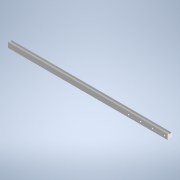
# Autodesk Inventor part: HSR35R128020 Rail
Saved by Autodesk Inventor 2022 (Build 260153000, 153)
## iProperties
Part Number: HSR35R128020 Rail
Material: Generic
Catalog Web Link: www.cadenas.de
Description: Compact Type - Heavy Load HSR-R Rail-Rail
Vendor: THK
Document SubType Name: Modeling
Designer: partserver
Manufacturer: THK
Mass: 224.938 g
Surface Area: 416.736 cm^2
Volume: 224.938 cm^3
Density: 1 g/cm^3
Appearance: PSOLRGB-192-192-192
Category: PARTsolutions
Company: THK
PSOL_IDENT_0: {$CADENAS_DATA\23d-libs\thk\linear_motion_systems\lm_guide\lm_guide\lm_guide_hsr\four_taped_hole_typ
PSOL_IDENT_1: e\hsr_r\hsr_r_rail.prj},219 {VTYP=3D},{NB=HSR35R128020 Rail},{LINA=HSR35R128020 Rail},{NN=Compact Ty
PSOL_IDENT_2: pe - Heavy Load HSR-R Rail},{DATE=21.06.2021 00:23:41},{GEOMDATE=24.12.2019 02:38:19},{VERSION=},{LI
PSOL_IDENT_3: NEID=70},{WBVAR=L,G,GX,TAPH},{WBNUMERIC=L,GX}  {NB=HSR35R128020 Rail},{LINA=HSR35R128020 Rail},{KT=D
PSOL_IDENT_4: UMMY},{MN=HSR35R},{NOB=1},{L=280.0},{G=},{GG='', 'Symmetrical (G1=G2)', 'A', 'Asymmetrical'},{GX=20}
PSOL_IDENT_5: ,{TAPH=},{GX1=20},{LMIN=109.4},{LEND=8640.00},{LMING=8.00},{LMAXG=32.00},{W1=34.00},{M1=29.00},{F=80
PSOL_IDENT_6: .00},{D1=9.00},{D2=14.00},{HM=12.00},{MAXL=3000.00},{GMIN=8},{GMX=20},{GMAX1=3.3},{G1=20},{G2=20},{N
PSOL_IDENT_7: X=1},{H3=7.50},{A=4},{LF=-20},{LM=320},{LL=620},{AA=3},{GMAX=32},{P=4},{PX=0},{VG=3},{VGG=20},{VG1=-
PSOL_IDENT_8: 1},{VG2=4},{ND=5.000},{LT=2880},{GA=20.000},{X=0.000},{S1=8.000},{L1=17.000},{NOTE=MIN}
NB: HSR35R128020 Rail
NN: Compact Type - Heavy Load HSR-R Rail
NT: Rail
NBSYN: $MN.$NOB.$L.$G.$GX.$TAPH. Rail
LINA: HSR35R128020 Rail
CATALOG: THK
MN: HSR35R
NOB: 1
L: 280
G: Symmetrical (G1=G2)
GX: 20
TAPH: Standard
LEND: 8640
LMING: 8
LMAXG: 32
W1: 34
M1: 29
F: 80
D1: 9
D2: 14
HM: 12
MAXL: 3000
H3: 7.5
ND: 5
GA: 20
X: 0
S1: 8
L1: 17
NOTE: 0
SUPPLIER: THK
ARTICLENO: HSR35R128020 Rail
BOMINFO: HSR35R128020 Rail
CREATOR: CADENAS GmbH
Title: HSR35R128020 Rail
Author: Cadenas PARTsolutions
Comments: Rail
Autodesk Inventor part; units mm, degrees
sketch "Sketch_18" plane through (-20, 0, 0) normal (1, 0, 0) x (0, 0, -1)
  line L0 (-17, 1.5) -> (-15.5, 0)
  line L1 (-15.5, 0) -> (-8.745, 0)
  line L2 (-8.745, 0) -> (-8.245, 0.5)
  line L3 (-8.245, 0.5) -> (-3.75, 0.5)
  line L4 (-3.75, 0.5) -> (-3.25, 0)
  line L5 (-3.25, 0) -> (3.25, 0)
  line L6 (3.25, 0) -> (3.75, 0.5)
  line L7 (3.75, 0.5) -> (8.245, 0.5)
  line L8 (8.245, 0.5) -> (8.745, 0)
  line L9 (8.745, 0) -> (15.5, 0)
  line L10 (15.5, 0) -> (17, 1.5)
  line L11 (17, 1.5) -> (17, 7.0002)
  line L12 (17, 7.0002) -> (11.8003, 12.1999)
  line L13 (11.8003, 12.1999) -> (11.8003, 17.6796)
  line L14 (11.8003, 17.6796) -> (13.6381, 19.5174)
  arc A0 (16.4816, 22.3609) -> (13.6381, 19.5174) centre (16.9102, 19.0889) ccw
  line L15 (16.4816, 22.3609) -> (17, 22.8793)
  line L16 (17, 22.8793) -> (17, 25.1102)
  line L17 (17, 25.1102) -> (16.4686, 25.6415)
  arc A1 (13.6398, 28.4703) -> (16.4686, 25.6415) centre (16.9102, 28.9119) ccw
  line L18 (13.6398, 28.4703) -> (13.1102, 29)
  line L19 (13.1102, 29) -> (-13.1102, 29)
  line L20 (-13.1102, 29) -> (-13.6398, 28.4703)
  arc A2 (-16.4686, 25.6415) -> (-13.6398, 28.4703) centre (-16.9102, 28.9119) ccw
  line L21 (-16.4686, 25.6415) -> (-17, 25.1102)
  line L22 (-17, 25.1102) -> (-17, 22.8793)
  line L23 (-17, 22.8793) -> (-16.4816, 22.3609)
  arc A3 (-13.6381, 19.5174) -> (-16.4816, 22.3609) centre (-16.9102, 19.0889) ccw
  line L24 (-13.6381, 19.5174) -> (-11.8003, 17.6796)
  line L25 (-11.8003, 17.6796) -> (-11.8003, 12.1999)
  line L26 (-11.8003, 12.1999) -> (-17, 7.0002)
  line L27 (-17, 7.0002) -> (-17, 1.5)
  constraints: 56 end point, 8 point on circle, 4 centre point
extrude "Extrusion1" add sketch "Sketch_18" along normal mid plane 1676.4
sketch "Sketch2" plane through (-858.2, 29, 13.1102) normal (0, 1, 0) x (1, 0, 0)
  point P0 (20, 13.1102)
hole "Hole1" at (-838.2, 29, 0) direction (0, -1, 0) diameter 9 depth 29 counterbore diameter 14 counterbore depth 12
pattern_linear "Rectangular Pattern1" count 4 spacing 80 along (1, 0, 0) of "Hole1"
ref_plane "4dummy_XY" through (0, 0, 0) normal (1, 0, 0) x (0, 0, -1)
ref_plane "4dummy_YZ" through (0, 0, 0) normal (0, 0, -1) x (0, 1, 0)
ref_plane "4dummy_ZX" through (0, 0, 0) normal (0, 1, 0) x (1, 0, 0)
ref_plane "4slide_XY" through (-20, 7.5, 0) normal (1, 0, 0) x (0, 0, -1)
ref_plane "4slide_YZ" through (-20, 7.5, 0) normal (0, 0, -1) x (0, 1, 0)
ref_plane "4slide_ZX" through (-20, 7.5, 0) normal (0, 1, 0) x (1, 0, 0)
ref_plane "4track_XY" through (0, 0, 0) normal (0, 0, 1) x (1, 0, 0)
ref_plane "4track_YZ" through (0, 0, 0) normal (1, 0, 0) x (0, 1, 0)
ref_plane "4track_ZX" through (0, 0, 0) normal (0, 1, 0) x (0, 0, 1)
body "Solid1"
